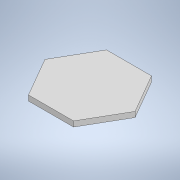
# Autodesk Inventor part: SatelliteTopFace_v2
Saved by Autodesk Inventor 2020 (Build 240168000, 168)
## iProperties
Created: 2020-03-05
Part Number: SatelliteTopFace_v2
Material: Generic
Document SubType Name: Modeling
Designer: WANG
Density: 1 g/cm^3
Appearance: Default
Author: WANG
Autodesk Inventor part; units mm, degrees
ref_plane "YZ Plane" through (0, 0, 0) normal (1, 0, 0) x (0, 1, 0)
ref_plane "XZ Plane" through (0, 0, 0) normal (0, 1, 0) x (-1, 0, 0)
ref_plane "XY Plane" through (0, 0, 0) normal (0, 0, 1) x (1, 0, 0)
sketch "Sketch1" plane through (0, 0, 0) normal (0, 1, 0) x (-1, 0, 0)
  line L0 (-107.95, 0) -> (-53.975, 93.4874)
  line L1 (-53.975, 93.4874) -> (53.975, 93.4874)
  line L2 (53.975, 93.4874) -> (107.95, 0)
  line L3 (107.95, 0) -> (53.975, -93.4874)
  line L4 (53.975, -93.4874) -> (-53.975, -93.4874)
  line L5 (-53.975, -93.4874) -> (-107.95, 0)
  line L6 (-95.25, 0.0344) -> (-47.5952, 82.5062)
  line L7 (-47.5952, 82.5062) -> (47.6548, 82.4717)
  line L8 (47.6548, 82.4717) -> (95.25, -0.0344)
  line L9 (95.25, -0.0344) -> (47.5952, -82.5062)
  line L10 (47.5952, -82.5062) -> (-47.6548, -82.4717)
  line L11 (-47.6548, -82.4717) -> (-95.25, 0.0344)
  point P0 (0, 0)
  point P1 (0, 0)
  point P2 (0, 0)
  dimension "d0" = 215.9
  dimension "d1" = 12.7
  constraints: 24 end point, 2 coincident, 26 other
  measures "d0" distance of L0.start L2.end
  measures "d1" distance of L0.start L6.start
extrude "Extrusion1" add sketch "Sketch1" along normal blind 12.7 contours L0 L1 L2 L3 L4 L5 | L6 L7 L8 L9 L10 L11
sketch "Sketch2" plane through (0, 0, 0) normal (0, -1, 0) x (1, 0, 0)
  line L0 (-107.95, -0.0034) -> (-53.9779, 93.4857)
  line L1 (-53.9779, 93.4857) -> (53.9721, 93.4891)
  line L2 (53.9721, 93.4891) -> (107.95, 0.0034)
  line L3 (107.95, 0.0034) -> (53.9779, -93.4857)
  line L4 (53.9779, -93.4857) -> (-53.9721, -93.4891)
  line L5 (-53.9721, -93.4891) -> (-107.95, -0.0034)
  line L6 (-92.964, 0.0336) -> (-46.4529, 80.526)
  line L7 (-46.4529, 80.526) -> (46.5111, 80.4924)
  line L8 (46.5111, 80.4924) -> (92.964, -0.0336)
  line L9 (92.964, -0.0336) -> (46.4529, -80.526)
  line L10 (46.4529, -80.526) -> (-46.5111, -80.4924)
  line L11 (-46.5111, -80.4924) -> (-92.964, 0.0336)
  point P0 (0, 0)
  point P1 (0, 0)
  point P2 (0, 0)
  point P3 (0, 0)
  point P4 (0, 0)
  dimension "d4" = 215.9
  dimension "d5" = 14.986
  constraints: 24 end point, 2 coincident, 26 other
  measures "d4" distance of L0.start L2.end
  measures "d5" distance of L0.start L6.start
extrude "Extrusion2" add sketch "Sketch2" along normal blind 6.35 contours L6 L7 L8 L9 L10 L11
sketch "Sketch3" plane through (0, 12.7, 0) normal (0, 1, 0) x (1, 0, 0)
  line L0 (-69.4244, 65.254) -> (70.2756, 65.254)
  line L1 (107.95, 0) -> (53.975, 93.4874) projected
  line L2 (-107.95, -0.0034) -> (-53.9779, 93.4857)
  line L3 (-53.9779, 93.4857) -> (53.9721, 93.4891)
  line L4 (53.9721, 93.4891) -> (107.95, 0.0034)
  line L5 (107.95, 0.0034) -> (53.9779, -93.4857)
  line L6 (53.9779, -93.4857) -> (-53.9721, -93.4891)
  line L7 (-53.9721, -93.4891) -> (-107.95, -0.0034)
  point P0 (0, 0)
  point P1 (0, 0)
  point P2 (0, 0)
  point P3 (0, 0)
  point P4 (0, 0)
  point P5 (0, 0)
  dimension "d8" = 139.7
  dimension "d9" = 215.9
  constraints: 14 end point, 2 coincident, 1 horizontal, 1 point on line, 13 other
  measures "d8" distance of L0.start L0.end
  measures "d9" distance of L2.start L4.end
body "Solid1"
